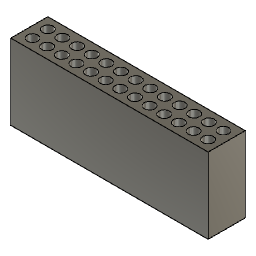
PTFE Sizing Template v1 (Autodesk Fusion 360 design; units mm, degrees)
Autodesk Fusion 360 part; units mm, degrees
sketch "Sketch1" plane through (0, 0, 0) normal (0, 0, 1) x (1, 0, 0)
  circle A0 centre (-50.4, 10) radius 2.25
  circle A1 centre (-50.4, 10) radius 1.9
  circle A2 centre (-44.2, 10) radius 1.9
  circle A3 centre (-44.2, 10) radius 2.25
  circle A4 centre (-38, 10) radius 1.9
  circle A5 centre (-38, 10) radius 2.25
  circle A6 centre (-31.8, 10) radius 1.9
  circle A7 centre (-31.8, 10) radius 2.25
  circle A8 centre (-25.6, 10) radius 1.9
  circle A9 centre (-25.6, 10) radius 2.25
  circle A10 centre (-19.4, 10) radius 1.9
  circle A11 centre (-19.4, 10) radius 2.25
  circle A12 centre (-13.2, 10) radius 1.9
  circle A13 centre (-13.2, 10) radius 2.25
  circle A14 centre (-7, 10) radius 1.9
  circle A15 centre (-7, 10) radius 2.25
  circle A16 centre (-0.8, 10) radius 1.9
  circle A17 centre (-0.8, 10) radius 2.25
  circle A18 centre (-31.8, 10) radius 1.9
  circle A19 centre (-25.6, 10) radius 1.9
  circle A20 centre (-38, 10) radius 1.9
  circle A21 centre (-7, 10) radius 1.9
  circle A22 centre (-19.4, 10) radius 1.9
  circle A23 centre (-0.8, 10) radius 1.9
  circle A24 centre (-13.2, 10) radius 1.9
  circle A25 centre (-44.2, 10) radius 1.9
  circle A26 centre (-50.4, 10) radius 1.9
  circle A27 centre (-31.8, 10) radius 1.9
  circle A28 centre (-25.6, 10) radius 1.9
  circle A29 centre (-38, 10) radius 1.9
  circle A30 centre (-7, 10) radius 1.9
  circle A31 centre (-19.4, 10) radius 1.9
  circle A32 centre (-0.8, 10) radius 1.9
  circle A33 centre (-13.2, 10) radius 1.9
  circle A34 centre (-44.2, 10) radius 1.9
  circle A35 centre (-50.4, 10) radius 1.9
  circle A36 centre (-25.6, 16.5) radius 1.9
  circle A37 centre (-44.2, 16.5) radius 1.9
  circle A38 centre (-0.8, 16.5) radius 1.9
  circle A39 centre (-31.8, 16.5) radius 1.9
  circle A40 centre (-50.4, 16.5) radius 1.9
  circle A41 centre (-19.4, 16.5) radius 1.9
  circle A42 centre (-44.2, 16.5) radius 1.9
  circle A43 centre (-0.8, 16.5) radius 2.25
  circle A44 centre (-31.8, 16.5) radius 1.9
  circle A45 centre (-13.2, 16.5) radius 1.9
  circle A46 centre (-38, 16.5) radius 1.9
  circle A47 centre (-19.4, 16.5) radius 1.9
  circle A48 centre (-50.4, 16.5) radius 1.9
  circle A49 centre (-31.8, 16.5) radius 1.9
  circle A50 centre (-0.8, 16.5) radius 1.9
  circle A51 centre (-44.2, 16.5) radius 2.25
  circle A52 centre (-25.6, 16.5) radius 1.9
  circle A53 centre (-50.4, 16.5) radius 1.9
  circle A54 centre (-31.8, 16.5) radius 2.25
  circle A55 centre (-38, 16.5) radius 2.25
  circle A56 centre (-38, 16.5) radius 1.9
  circle A57 centre (-7, 16.5) radius 1.9
  circle A58 centre (-7, 16.5) radius 1.9
  circle A59 centre (-7, 16.5) radius 2.25
  circle A60 centre (-7, 16.5) radius 1.9
  circle A61 centre (-19.4, 16.5) radius 1.9
  circle A62 centre (-0.8, 16.5) radius 1.9
  circle A63 centre (-38, 16.5) radius 1.9
  circle A64 centre (-13.2, 16.5) radius 1.9
  circle A65 centre (-13.2, 16.5) radius 2.25
  circle A66 centre (-44.2, 16.5) radius 1.9
  circle A67 centre (-25.6, 16.5) radius 1.9
  circle A68 centre (-19.4, 16.5) radius 2.25
  circle A69 centre (-25.6, 16.5) radius 2.25
  circle A70 centre (-50.4, 16.5) radius 2.25
  circle A71 centre (-13.2, 16.5) radius 1.9
  line L0 (-55, 5.4) -> (-55, 21.1)
  circle A72 centre (5.4, 10) radius 1.9
  circle A73 centre (5.4, 10) radius 2.25
  circle A74 centre (5.4, 16.5) radius 2.25
  circle A75 centre (5.4, 16.5) radius 1.9
  circle A76 centre (11.6, 10) radius 1.9
  circle A77 centre (11.6, 10) radius 2.25
  circle A78 centre (11.6, 16.5) radius 2.25
  circle A79 centre (11.6, 16.5) radius 1.9
  circle A80 centre (17.8, 10) radius 1.9
  circle A81 centre (17.8, 10) radius 2.25
  circle A82 centre (17.8, 16.5) radius 2.25
  circle A83 centre (17.8, 16.5) radius 1.9
  circle A84 centre (24, 10) radius 1.9
  circle A85 centre (24, 10) radius 2.25
  circle A86 centre (24, 16.5) radius 2.25
  circle A87 centre (24, 16.5) radius 1.9
  line L1 (28.6, 21.1) -> (28.6, 5.4)
  line L2 (-55, 5.4) -> (28.6, 5.4)
  line L3 (-55, 21.1) -> (28.6, 21.1)
  point P0 (0, 6.5)
  dimension "d3" = 4.5
  dimension "d5" = 3.8
  dimension "d12" = 6.2
  dimension "d13" = 0
  dimension "d43" = 3.8
  dimension "d53" = 3.8
  dimension "d63" = 6.2
  dimension "d64" = 0
  dimension "d70" = 4.6
  dimension "d71" = 3.8
  dimension "d75" = 4.5
  dimension "d77" = 3.8
  dimension "d83" = 3.8
  dimension "d133" = 4.6
  dimension "d169" = 4.5
  dimension "d170" = 4.5
  dimension "d171" = 4.5
  dimension "d172" = 4.5
  dimension "d173" = 4.5
  dimension "d174" = 4.5
  dimension "d175" = 4.5
  dimension "d176" = 4.5
  dimension "d177" = 4.5
  constraint concentric A0 A1
  constraint vertical L0
  constraint concentric A40 A70
  constraint perpendicular L1 L3
  measures "d3" diameter of A0
  measures "d5" diameter of A1
  measures "d43" diameter of A26
  measures "d53" diameter of A35
  measures "d70" distance of A40.centre L0
  measures "d71" diameter of A53
  measures "d75" diameter of A70
  measures "d77" diameter of A40
  measures "d83" diameter of A48
  measures "d133" distance of A86.centre L1
  measures "d169" diameter of A43
  measures "d170" diameter of A73
  measures "d171" diameter of A74
  measures "d172" diameter of A77
  measures "d173" diameter of A78
  measures "d174" diameter of A82
  measures "d175" diameter of A81
  measures "d176" diameter of A85
  measures "d177" diameter of A86
extrude "Extrude11" add sketch "Sketch1" along normal blind 32 contours L0 L1 L2 L3 | A72 | A73 | A74 | A75 | A76 | A77 | A78 | A79 | A80 | A81 | A82 | A83 | A84 | A85 | A86 | A87
extrude "Extrude12" add sketch "Sketch1" along normal blind 2.2 contours A0
extrude "Extrude13" add sketch "Sketch1" along normal blind 3.4 contours A3
extrude "Extrude14" add sketch "Sketch1" along normal blind 4 contours A5
extrude "Extrude15" add sketch "Sketch1" along normal blind 5 contours A7
extrude "Extrude16" add sketch "Sketch1" along normal blind 6.4 contours A9
extrude "Extrude17" add sketch "Sketch1" along normal blind 7 contours A11
extrude "Extrude18" add sketch "Sketch1" along normal blind 8 contours A13
extrude "Extrude19" add sketch "Sketch1" along normal blind 9.2 contours A15
extrude "Extrude20" add sketch "Sketch1" along normal blind 9.35 contours A17
extrude "Extrude30" cut sketch "Sketch1" along normal blind 33 contours A16 A23 A32 | A17 | A38 A50 A62 | A43 | A72 | A73 | A74 | A75 | A76 | A77 | A78 | A79 | A80 | A81 | A82 | A83 | A84 | A85 | A86 | A87
extrude "Extrude31" add sketch "Sketch1" along normal blind 10.4 contours A17
extrude "Extrude32" add sketch "Sketch1" along normal blind 11.26 contours A73
extrude "Extrude33" add sketch "Sketch1" along normal blind 12.3 contours A77
extrude "Extrude34" add sketch "Sketch1" along normal blind 13.1 contours A81
extrude "Extrude35" add sketch "Sketch1" along normal blind 14.1 contours A85
extrude "Extrude21" add sketch "Sketch1" along normal blind 15.3 contours A70
extrude "Extrude22" add sketch "Sketch1" along normal blind 16.35 contours A51
extrude "Extrude46" add sketch "Sketch1" along normal blind 17.45 contours A55
extrude "Extrude36" add sketch "Sketch1" along normal blind 18.35 contours A54
extrude "Extrude37" add sketch "Sketch1" along normal blind 19.35 contours A69
extrude "Extrude38" add sketch "Sketch1" along normal blind 20.25 contours A68
extrude "Extrude39" add sketch "Sketch1" along normal blind 21.35 contours A65
extrude "Extrude40" add sketch "Sketch1" along normal blind 22.3 contours A59
extrude "Extrude41" add sketch "Sketch1" along normal blind 23.65 contours A43
extrude "Extrude42" add sketch "Sketch1" along normal blind 24.65 contours A74
extrude "Extrude43" add sketch "Sketch1" along normal blind 25.3 contours A78
extrude "Extrude44" add sketch "Sketch1" along normal blind 26.3 contours A82
extrude "Extrude45" add sketch "Sketch1" along normal blind 27.25 contours A86
extrude "Extrude23" [suppressed]
extrude "Extrude24" [suppressed]
extrude "Extrude25" [suppressed]
extrude "Extrude26" [suppressed]
extrude "Extrude27" [suppressed]
extrude "Extrude28" [suppressed]
extrude "Extrude29" [suppressed]
extrude "Extrude1" [suppressed]
extrude "Extrude2" [suppressed]
extrude "Extrude3" [suppressed]
extrude "Extrude4" [suppressed]
extrude "Extrude5" [suppressed]
extrude "Extrude6" [suppressed]
extrude "Extrude7" [suppressed]
extrude "Extrude8" [suppressed]
extrude "Extrude9" [suppressed]
extrude "Extrude10" [suppressed]
equation "d3 = od_ptfe"
equation "d75 = od_ptfe"
equation "od_ptfe = 4.5 mm"
equation "d169 = od_ptfe"
equation "d170 = od_ptfe"
equation "d171 = od_ptfe"
equation "d172 = od_ptfe"
equation "d173 = od_ptfe"
equation "d174 = od_ptfe"
equation "d175 = od_ptfe"
equation "d176 = od_ptfe"
equation "d177 = od_ptfe"
named bodies: "PTFE Length Template"
